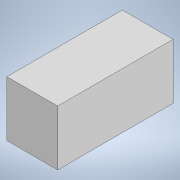
# Autodesk Inventor part: FS2A
Saved by Autodesk Inventor 2020 (Build 240168000, 168)
## iProperties
Created: 2023-12-14
Part Number: FS2A
Material: Generic
Document SubType Name: Modeling
Designer: smz3rm
Mass: 1 g
Surface Area: 14.14 cm^2
Volume: 3.3 cm^3
Density: 0.30303 g/cm^3
Appearance: Default
Author: smz3rm
Autodesk Inventor part; units mm, degrees
ref_plane "YZ Plane" through (0, 0, 0) normal (1, 0, 0) x (0, 1, 0)
ref_plane "XZ Plane" through (0, 0, 0) normal (0, 1, 0) x (-1, 0, 0)
ref_plane "XY Plane" through (0, 0, 0) normal (0, 0, 1) x (1, 0, 0)
sketch "Sketch1" plane through (0, 0, 0) normal (0, 1, 0) x (-1, 0, 0)
  line L0 (5.5, 12.5) -> (-5.5, 12.5)
  line L1 (-5.5, 12.5) -> (-5.5, -12.5)
  line L2 (-5.5, -12.5) -> (5.5, -12.5)
  line L3 (5.5, -12.5) -> (5.5, 12.5)
  line L4 (5.5, 12.5) -> (-5.5, -12.5) construction
  line L5 (-5.5, 12.5) -> (5.5, -12.5) construction
  point P0 (0, 0)
  dimension "d0" = 11
  dimension "d1" = 25
  constraints: 12 end point, 2 midpoint, 2 parallel, 1 horizontal, 1 perpendicular
  measures "d0" distance of L2.end L1.end
  measures "d1" distance of L1.end L0.end
extrude "Extrusion1" add sketch "Sketch1" along normal blind 12
body "Solid1"
